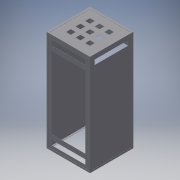
# Autodesk Inventor part: Cabinet_3x3x7
Saved by Autodesk Inventor 2017 (Build 210142000, 142)
## iProperties
Created: 2015-04-30
Part Number: Cabinet_3x3x7
Material: Generic
Document SubType Name: Modeling
Designer: mcgratta
Density: 1 g/cm^3
Appearance: Default
Author: mcgratta
Autodesk Inventor part; units mm, degrees
ref_plane "YZ Plane" through (0, 0, 0) normal (1, 0, 0) x (0, 1, 0)
ref_plane "XZ Plane" through (0, 0, 0) normal (0, 1, 0) x (-1, 0, 0)
ref_plane "XY Plane" through (0, 0, 0) normal (0, 0, 1) x (1, 0, 0)
sketch "Sketch1" plane through (0, 0, 0) normal (0, 1, 0) x (-1, 0, 0)
  line L0 (0, 0) -> (-920.75, 0)
  line L1 (-920.75, 0) -> (-920.75, -920.75)
  line L2 (-920.75, -920.75) -> (0, -920.75)
  line L3 (0, -920.75) -> (0, 0)
  line L4 (-38.1, -38.1) -> (-882.65, -38.1)
  line L5 (-882.65, -38.1) -> (-882.65, -882.65)
  line L6 (-882.65, -882.65) -> (-38.1, -882.65)
  line L7 (-38.1, -882.65) -> (-38.1, -38.1)
  dimension "d0" = 920.75
  dimension "d3" = 920.75
  dimension "d4" = 38.1
  dimension "d5" = 38.1
  dimension "d6" = 38.1
  dimension "d7" = 38.1
  constraints: 16 end point, 4 parallel, 2 horizontal, 2 perpendicular
  measures "d0" distance between parallel lines of L1 L3
  measures "d3" distance between parallel lines of L0 L2
  measures "d4" distance between parallel lines of L0 L4
  measures "d5" distance between parallel lines of L3 L7
  measures "d6" distance between parallel lines of L2 L6
  measures "d7" distance between parallel lines of L1 L5
extrude "Extrusion1" add sketch "Sketch1" along normal blind 3.175
sketch "Sketch2" plane through (0, 3.175, 0) normal (0, 1, 0) x (1, 0, 0)
  line L0 (0, 0) -> (920.75, 0) projected
  line L1 (920.75, 0) -> (920.75, 920.75) projected
  line L2 (920.75, 920.75) -> (0, 920.75) projected
  line L3 (0, 0) -> (920.75, 0)
  line L4 (920.75, 0) -> (920.75, 920.75)
  line L5 (920.75, 920.75) -> (0, 920.75)
  line L6 (0, 920.75) -> (0, 0)
  line L7 (3.175, 3.175) -> (917.575, 3.175)
  line L8 (917.575, 3.175) -> (917.575, 917.575)
  line L9 (917.575, 917.575) -> (3.175, 917.575)
  line L10 (3.175, 917.575) -> (3.175, 3.175)
  dimension "d10" = 3.175
  dimension "d12" = 3.175
  dimension "d13" = 3.175
  dimension "d14" = 3.175
  constraints: 16 end point, 4 parallel, 2 horizontal, 2 perpendicular
  measures "d10" distance between parallel lines of L10 L6
  measures "d12" distance between parallel lines of L9 L2
  measures "d13" distance between parallel lines of L1 L8
  measures "d14" distance between parallel lines of L0 L7
extrude "Extrusion2" add sketch "Sketch2" along normal blind 34.925
sketch "Sketch3" plane through (0, 38.1, 0) normal (0, 1, 0) x (1, 0, 0)
  line L0 (3.175, 3.175) -> (3.175, 917.575) projected
  line L1 (917.575, 917.575) -> (917.575, 3.175) projected
  line L2 (917.575, 3.175) -> (3.175, 3.175) projected
  line L3 (0, 0) -> (920.75, 0) projected
  line L4 (920.75, 0) -> (920.75, 920.75) projected
  line L5 (0, 920.75) -> (0, 0) projected
  line L6 (0, 0) -> (38.1, 0)
  line L7 (38.1, 3.175) -> (3.175, 3.175)
  line L8 (3.175, 38.1) -> (0, 38.1)
  line L9 (38.1, 0) -> (38.1, 3.175)
  line L10 (920.75, 0) -> (920.75, 38.1)
  line L11 (917.575, 38.1) -> (917.575, 3.175)
  line L12 (882.65, 3.175) -> (882.65, 0)
  line L13 (917.575, 38.1) -> (920.75, 38.1)
  dimension "d17" = 38.1
  dimension "d18" = 38.1
  dimension "d19" = 38.1
  dimension "d20" = 38.1
  dimension "d21" = 38.1
  dimension "d22" = 38.1
  constraints: 16 end point, 8 point on line, 2 collinear, 2 perpendicular
  measures "d17" distance between parallel lines of L6 L8
  measures "d18" distance from line of L6.end L5
  measures "d19" distance from line of L7.start L5
  measures "d20" distance between parallel lines of L4 L12
  measures "d21" distance from line of L11.start L3
  measures "d22" distance from line of L3 L10.end
extrude "Extrusion3" add sketch "Sketch3" along normal blind 2063.75 contours L2 L9 L3 L5 L8 L0 | L2 L1 L13 L4 L3 L12
sketch "Sketch4" plane through (0, 38.1, 0) normal (0, 1, 0) x (1, 0, 0)
  line L0 (3.175, 38.1) -> (3.175, 917.575) projected
  line L1 (3.175, 917.575) -> (917.575, 917.575) projected
  line L2 (917.575, 917.575) -> (917.575, 38.1) projected
  line L3 (920.75, 38.1) -> (920.75, 920.75) projected
  line L4 (920.75, 920.75) -> (0, 920.75) projected
  line L5 (0, 920.75) -> (0, 38.1) projected
  line L6 (0, 920.75) -> (0, 882.65)
  line L7 (3.175, 882.65) -> (3.175, 917.575)
  line L8 (38.1, 917.575) -> (38.1, 920.75)
  line L9 (0, 882.65) -> (3.175, 882.65)
  line L10 (920.75, 920.75) -> (882.65, 920.75)
  line L11 (882.65, 917.575) -> (917.575, 917.575)
  line L12 (917.575, 882.65) -> (920.75, 882.65)
  line L13 (882.65, 920.75) -> (882.65, 917.575)
  point P0 (0, 0)
  dimension "d25" = 38.1
  dimension "d26" = 38.1
  dimension "d27" = 38.1
  dimension "d28" = 38.1
  constraints: 16 end point, 8 point on line, 4 perpendicular, 2 collinear
  measures "d25" distance between parallel lines of L8 L6
  measures "d26" distance from line of L4 L6.end
  measures "d27" distance between parallel lines of L3 L13
  measures "d28" distance between parallel lines of L12 L4
extrude "Extrusion4" add sketch "Sketch4" along normal blind 2063.75 contours L9 L5 L4 L8 L1 L0 | L13 L4 L3 L12 L2 L1
sketch "Sketch5" plane through (0, 3.175, 0) normal (0, 1, 0) x (1, 0, 0)
  line L0 (3.175, 3.175) -> (917.575, 3.175) projected
  line L1 (3.175, 3.175) -> (917.575, 3.175)
  line L2 (917.575, 3.175) -> (917.575, 917.575)
  line L3 (917.575, 917.575) -> (3.175, 917.575)
  line L4 (3.175, 917.575) -> (3.175, 3.175)
  line L5 (5.8318, 5.8318) -> (914.9182, 5.8318)
  line L6 (914.9182, 5.8318) -> (914.9182, 914.9182)
  line L7 (914.9182, 914.9182) -> (5.8318, 914.9182)
  line L8 (5.8318, 914.9182) -> (5.8318, 5.8318)
  point P0 (0, 0)
  dimension "d31" = 914.4
  dimension "d33" = 914.4
  dimension "d34" = 2.6568
  dimension "d35" = 2.6568
  dimension "d36" = 909.0863
  dimension "d37" = 909.0863
  constraints: 16 end point, 4 parallel, 2 horizontal, 2 perpendicular
  measures "d31" distance between parallel lines of L2 L4
  measures "d33" distance between parallel lines of L0 L3
  measures "d34" distance between parallel lines of L8 L4
  measures "d35" distance between parallel lines of L1 L5
  measures "d36" distance between parallel lines of L5 L7
  measures "d37" distance between parallel lines of L6 L8
extrude "Extrusion5" add sketch "Sketch5" along normal blind 2133.6
sketch "Sketch6" plane through (0, 2101.85, 0) normal (0, 1, 0) x (1, 0, 0)
  line L0 (920.75, 0) -> (0, 0)
  line L1 (0, 0) -> (0, 920.75)
  line L2 (0, 920.75) -> (920.75, 920.75)
  line L3 (920.75, 920.75) -> (920.75, 0)
  line L4 (917.575, 3.175) -> (3.175, 3.175)
  line L5 (3.175, 3.175) -> (3.175, 917.575)
  line L6 (3.175, 917.575) -> (917.575, 917.575)
  line L7 (917.575, 917.575) -> (917.575, 3.175)
  point P0 (0, 0)
  dimension "d40" = 920.75
  dimension "d42" = 920.75
  dimension "d43" = 914.4
  dimension "d44" = 914.4
  constraints: 16 end point, 4 parallel, 2 horizontal, 2 perpendicular
  measures "d40" distance between parallel lines of L3 L1
  measures "d42" distance between parallel lines of L0 L2
  measures "d43" distance between parallel lines of L4 L6
  measures "d44" distance between parallel lines of L5 L7
extrude "Extrusion6" add sketch "Sketch6" along normal blind 38.1
sketch "Sketch7" plane through (0, 2136.775, 0) normal (0, 1, 0) x (1, 0, 0)
  line L0 (5.8318, 5.8318) -> (5.8318, 914.9182) projected
  line L1 (5.8318, 914.9182) -> (914.9182, 914.9182) projected
  line L2 (914.9182, 914.9182) -> (914.9182, 5.8318) projected
  line L3 (914.9182, 5.8318) -> (5.8318, 5.8318) projected
  line L4 (5.8318, 5.8318) -> (914.9182, 5.8318)
  line L5 (914.9182, 5.8318) -> (914.9182, 914.9182)
  line L6 (914.9182, 914.9182) -> (5.8318, 914.9182)
  line L7 (5.8318, 914.9182) -> (5.8318, 5.8318)
  point P0 (0, 0)
  dimension "d47" = 909.0863
  dimension "d49" = 909.0863
  constraints: 8 end point, 2 parallel, 1 horizontal, 1 perpendicular
  measures "d47" distance between parallel lines of L5 L7
  measures "d49" distance between parallel lines of L6 L3
extrude "Extrusion7" add sketch "Sketch7" against normal blind 3.175
sketch "Sketch8" plane through (0, 2136.775, 0) normal (0, 1, 0) x (1, 0, 0)
  line L0 (3.175, 3.175) -> (917.575, 3.175) projected
  line L1 (917.575, 3.175) -> (917.575, 917.575) projected
  line L2 (917.575, 917.575) -> (3.175, 917.575) projected
  line L3 (3.175, 917.575) -> (3.175, 3.175) projected
  line L4 (3.175, 3.175) -> (917.575, 3.175)
  line L5 (917.575, 3.175) -> (917.575, 917.575)
  line L6 (917.575, 917.575) -> (3.175, 917.575)
  line L7 (3.175, 917.575) -> (3.175, 3.175)
  line L8 (38.1, 38.1) -> (882.65, 38.1)
  line L9 (882.65, 38.1) -> (882.65, 882.65)
  line L10 (882.65, 882.65) -> (38.1, 882.65)
  line L11 (38.1, 882.65) -> (38.1, 38.1)
  point P0 (0, 0)
  dimension "d52" = 914.4
  dimension "d54" = 914.4
  dimension "d55" = 34.925
  dimension "d56" = 34.925
  dimension "d57" = 844.55
  dimension "d58" = 844.55
  constraints: 16 end point, 4 parallel, 2 horizontal, 2 perpendicular
  measures "d52" distance between parallel lines of L4 L6
  measures "d54" distance between parallel lines of L5 L3
  measures "d55" distance between parallel lines of L11 L3
  measures "d56" distance between parallel lines of L0 L8
  measures "d57" distance between parallel lines of L9 L11
  measures "d58" distance between parallel lines of L8 L10
extrude "Extrusion8" add sketch "Sketch8" along normal blind 3.175
sketch "Sketch9" plane through (38.1, 38.1, -3.175) normal (0, 0, 1) x (1, 0, 0)
  line L0 (844.55, 2063.75) -> (0, 2063.75) projected
  line L1 (0, 0) -> (0, 2063.75) projected
  line L2 (844.55, 0) -> (0, 0) projected
  line L3 (844.55, 0) -> (844.55, 2063.75) projected
  line L4 (63.5, 2000.25) -> (781.05, 2000.25)
  line L5 (781.05, 2000.25) -> (781.05, 1898.65)
  line L6 (781.05, 1898.65) -> (63.5, 1898.65)
  line L7 (63.5, 1898.65) -> (63.5, 2000.25)
  line L8 (63.5, 1797.05) -> (781.05, 1797.05)
  line L9 (781.05, 1797.05) -> (781.05, 266.7)
  line L10 (781.05, 266.7) -> (63.5, 266.7)
  line L11 (63.5, 266.7) -> (63.5, 1797.05)
  line L12 (63.5, 165.1) -> (781.05, 165.1)
  line L13 (781.05, 165.1) -> (781.05, 63.5)
  line L14 (781.05, 63.5) -> (63.5, 63.5)
  line L15 (63.5, 63.5) -> (63.5, 165.1)
  point P0 (-38.1, -38.1)
  dimension "d61" = 63.5
  dimension "d62" = 0
  dimension "d63" = 0
  dimension "d64" = 63.5
  dimension "d65" = 101.6
  dimension "d66" = 63.5
  dimension "d67" = 101.6
  dimension "d68" = 101.6
  dimension "d69" = 101.6
  dimension "d70" = 63.5
  dimension "d71" = 0
  dimension "d72" = 0
  constraints: 24 end point, 6 parallel, 3 horizontal, 3 perpendicular
  measures "d61" distance between parallel lines of L7 L1
  measures "d62" distance between parallel lines of L11 L7
  measures "d63" distance between parallel lines of L15 L11
  measures "d64" distance between parallel lines of L4 L0
  measures "d65" distance between parallel lines of L8 L6
  measures "d66" distance between parallel lines of L14 L2
  measures "d67" distance between parallel lines of L14 L12
  measures "d68" distance between parallel lines of L12 L10
  measures "d69" distance between parallel lines of L6 L4
  measures "d70" distance between parallel lines of L3 L5
  measures "d71" distance between parallel lines of L9 L5
  measures "d72" distance between parallel lines of L9 L13
extrude "Extrusion9" cut sketch "Sketch9" against normal blind 2.6568 contours L4 L5 L6 L7 | L8 L9 L10 L11 | L12 L13 L14 L15
sketch "Sketch10" plane through (882.65, 38.1, -917.575) normal (0, 0, -1) x (-1, 0, 0)
  line L0 (844.55, 2063.75) -> (0, 2063.75) projected
  line L1 (0, 0) -> (0, 2063.75) projected
  line L2 (844.55, 0) -> (0, 0) projected
  line L3 (844.55, 0) -> (844.55, 2063.75) projected
  line L4 (63.5, 2000.25) -> (781.05, 2000.25)
  line L5 (781.05, 2000.25) -> (781.05, 1898.65)
  line L6 (781.05, 1898.65) -> (63.5, 1898.65)
  line L7 (63.5, 1898.65) -> (63.5, 2000.25)
  line L8 (63.5, 1797.05) -> (781.05, 1797.05)
  line L9 (781.05, 1797.05) -> (781.05, 266.7)
  line L10 (781.05, 266.7) -> (63.5, 266.7)
  line L11 (63.5, 266.7) -> (63.5, 1797.05)
  line L12 (63.5, 165.1) -> (781.05, 165.1)
  line L13 (781.05, 165.1) -> (781.05, 63.5)
  line L14 (781.05, 63.5) -> (63.5, 63.5)
  line L15 (63.5, 63.5) -> (63.5, 165.1)
  point P0 (882.65, -38.1)
  dimension "d75" = 63.5
  dimension "d76" = 63.5
  dimension "d77" = 63.5
  dimension "d78" = 101.6
  dimension "d79" = 101.6
  dimension "d80" = 0
  dimension "d81" = 0
  dimension "d82" = 101.6
  dimension "d83" = 101.6
  dimension "d84" = 63.5
  dimension "d85" = 0
  dimension "d86" = 0
  constraints: 24 end point, 6 parallel, 3 horizontal, 3 perpendicular
  measures "d75" distance between parallel lines of L7 L1
  measures "d76" distance between parallel lines of L3 L5
  measures "d77" distance between parallel lines of L4 L0
  measures "d78" distance between parallel lines of L6 L4
  measures "d79" distance between parallel lines of L8 L6
  measures "d80" distance between parallel lines of L11 L7
  measures "d81" distance between parallel lines of L15 L11
  measures "d82" distance between parallel lines of L12 L10
  measures "d83" distance between parallel lines of L14 L12
  measures "d84" distance between parallel lines of L2 L14
  measures "d85" distance between parallel lines of L5 L9
  measures "d86" distance between parallel lines of L13 L9
extrude "Extrusion10" cut sketch "Sketch10" against normal blind 2.6568 contours L4 L5 L6 L7 | L8 L9 L10 L11 | L12 L13 L14 L15
sketch "Sketch11" plane through (917.575, 38.1, -38.1) normal (1, 0, 0) x (0, 0, -1)
  line L0 (844.55, 2063.75) -> (0, 2063.75) projected
  line L1 (0, 0) -> (0, 2063.75) projected
  line L2 (844.55, 0) -> (844.55, 2063.75) projected
  line L3 (63.5, 2000.25) -> (781.05, 2000.25)
  line L4 (781.05, 2000.25) -> (781.05, 1898.65)
  line L5 (781.05, 1898.65) -> (63.5, 1898.65)
  line L6 (63.5, 1898.65) -> (63.5, 2000.25)
  point P0 (-38.1, -38.1)
  dimension "d89" = 63.5
  dimension "d90" = 63.5
  dimension "d91" = 63.5
  dimension "d92" = 101.6
  constraints: 8 end point, 2 parallel, 1 horizontal, 1 perpendicular
  measures "d89" distance between parallel lines of L6 L1
  measures "d90" distance between parallel lines of L3 L0
  measures "d91" distance between parallel lines of L4 L2
  measures "d92" distance between parallel lines of L5 L3
extrude "Extrusion11" cut sketch "Sketch11" against normal blind 2.6568
sketch "Sketch12" plane through (3.175, 38.1, -882.65) normal (-1, 0, 0) x (0, 0, 1)
  line L0 (844.55, 2063.75) -> (0, 2063.75) projected
  line L1 (0, 0) -> (0, 2063.75) projected
  line L2 (844.55, 0) -> (844.55, 2063.75) projected
  line L3 (63.5, 2000.25) -> (781.05, 2000.25)
  line L4 (781.05, 2000.25) -> (781.05, 1898.65)
  line L5 (781.05, 1898.65) -> (63.5, 1898.65)
  line L6 (63.5, 1898.65) -> (63.5, 2000.25)
  point P0 (882.65, -38.1)
  dimension "d95" = 63.5
  dimension "d96" = 63.5
  dimension "d97" = 63.5
  dimension "d98" = 101.6
  constraints: 8 end point, 2 parallel, 1 horizontal, 1 perpendicular
  measures "d95" distance between parallel lines of L6 L1
  measures "d96" distance between parallel lines of L3 L0
  measures "d97" distance between parallel lines of L4 L2
  measures "d98" distance between parallel lines of L5 L3
extrude "Extrusion12" cut sketch "Sketch12" against normal blind 2.6568
sketch "Sketch13" plane through (0, 2136.775, 0) normal (0, 1, 0) x (1, 0, 0)
  line L0 (920.75, 920.75) -> (0, 920.75) projected
  line L1 (0, 920.75) -> (0, 0) projected
  line L2 (409.575, 511.175) -> (511.175, 511.175)
  line L3 (511.175, 511.175) -> (511.175, 409.575)
  line L4 (511.175, 409.575) -> (409.575, 409.575)
  line L5 (409.575, 409.575) -> (409.575, 511.175)
  line L6 (0, 0) -> (920.75, 0) projected
  line L7 (612.775, 511.175) -> (714.375, 511.175)
  line L8 (714.375, 511.175) -> (714.375, 409.575)
  line L9 (714.375, 409.575) -> (612.775, 409.575)
  line L10 (612.775, 409.575) -> (612.775, 511.175)
  line L11 (206.375, 511.175) -> (307.975, 511.175)
  line L12 (307.975, 511.175) -> (307.975, 409.575)
  line L13 (307.975, 409.575) -> (206.375, 409.575)
  line L14 (206.375, 409.575) -> (206.375, 511.175)
  line L15 (409.575, 714.375) -> (511.175, 714.375)
  line L16 (511.175, 714.375) -> (511.175, 612.775)
  line L17 (511.175, 612.775) -> (409.575, 612.775)
  line L18 (409.575, 612.775) -> (409.575, 714.375)
  line L19 (612.775, 714.375) -> (714.375, 714.375)
  line L20 (714.375, 714.375) -> (714.375, 612.775)
  line L21 (714.375, 612.775) -> (612.775, 612.775)
  line L22 (612.775, 612.775) -> (612.775, 714.375)
  line L23 (206.375, 714.375) -> (307.975, 714.375)
  line L24 (307.975, 714.375) -> (307.975, 612.775)
  line L25 (307.975, 612.775) -> (206.375, 612.775)
  line L26 (206.375, 612.775) -> (206.375, 714.375)
  line L27 (409.575, 307.975) -> (511.175, 307.975)
  line L28 (511.175, 307.975) -> (511.175, 206.375)
  line L29 (511.175, 206.375) -> (409.575, 206.375)
  line L30 (409.575, 206.375) -> (409.575, 307.975)
  line L31 (612.775, 307.975) -> (714.375, 307.975)
  line L32 (714.375, 307.975) -> (714.375, 206.375)
  line L33 (714.375, 206.375) -> (612.775, 206.375)
  line L34 (612.775, 206.375) -> (612.775, 307.975)
  line L35 (206.375, 307.975) -> (307.975, 307.975)
  line L36 (307.975, 307.975) -> (307.975, 206.375)
  line L37 (307.975, 206.375) -> (206.375, 206.375)
  line L38 (206.375, 206.375) -> (206.375, 307.975)
  dimension "d150" = 409.575
  dimension "d151" = 101.6
  dimension "d152" = 409.575
  dimension "d153" = 101.6
  dimension "d154" = 101.6
  dimension "d155" = 101.6
  dimension "d156" = 101.6
  dimension "d157" = 101.6
  dimension "d158" = 101.6
  dimension "d159" = 101.6
  dimension "d160" = 101.6
  dimension "d161" = 101.6
  dimension "d162" = 101.6
  dimension "d163" = 101.6
  dimension "d164" = 101.6
  dimension "d165" = 101.6
  dimension "d166" = 101.6
  dimension "d167" = 101.6
  dimension "d168" = 101.6
  dimension "d169" = 101.6
  dimension "d170" = 101.6
  dimension "d171" = 101.6
  dimension "d172" = 101.6
  dimension "d173" = 101.6
  dimension "d174" = 101.6
  dimension "d175" = 101.6
  dimension "d176" = 101.6
  dimension "d177" = 101.6
  dimension "d178" = 101.6
  dimension "d179" = 101.6
  dimension "d180" = 101.6
  dimension "d181" = 101.6
  dimension "d182" = 101.6
  dimension "d183" = 101.6
  dimension "d184" = 101.6
  dimension "d185" = 101.6
  constraints: 72 end point, 18 parallel, 9 horizontal, 9 perpendicular
  measures "d150" distance between parallel lines of L5 L1
  measures "d151" distance between parallel lines of L3 L5
  measures "d152" distance between parallel lines of L6 L4
  measures "d153" distance between parallel lines of L4 L2
  measures "d154" distance between parallel lines of L10 L3
  measures "d155" distance between parallel lines of L9 L7
  measures "d156" distance between parallel lines of L2 L9
  measures "d157" distance between parallel lines of L8 L10
  measures "d158" distance between parallel lines of L13 L11
  measures "d159" distance between parallel lines of L12 L14
  measures "d160" distance between parallel lines of L5 L12
  measures "d161" distance between parallel lines of L4 L11
  measures "d162" distance between parallel lines of L16 L18
  measures "d163" distance between parallel lines of L17 L15
  measures "d164" distance between parallel lines of L22 L16
  measures "d165" distance between parallel lines of L21 L19
  measures "d166" distance between parallel lines of L15 L21
  measures "d167" distance between parallel lines of L20 L22
  measures "d168" distance between parallel lines of L25 L23
  measures "d169" distance between parallel lines of L24 L26
  measures "d170" distance between parallel lines of L18 L24
  measures "d171" distance between parallel lines of L17 L23
  measures "d172" distance between parallel lines of L28 L30
  measures "d173" distance between parallel lines of L29 L27
  measures "d174" distance between parallel lines of L34 L28
  measures "d175" distance between parallel lines of L33 L31
  measures "d176" distance between parallel lines of L27 L33
  measures "d177" distance between parallel lines of L32 L34
  measures "d178" distance between parallel lines of L37 L35
  measures "d179" distance between parallel lines of L36 L38
  measures "d180" distance between parallel lines of L30 L36
  measures "d181" distance between parallel lines of L29 L35
  measures "d182" distance between parallel lines of L11 L25
  measures "d183" distance between parallel lines of L18 L12
  measures "d184" distance between parallel lines of L35 L13
  measures "d185" distance between parallel lines of L5 L36
extrude "Extrusion13" cut sketch "Sketch13" against normal blind 3.175
body "Solid1"
